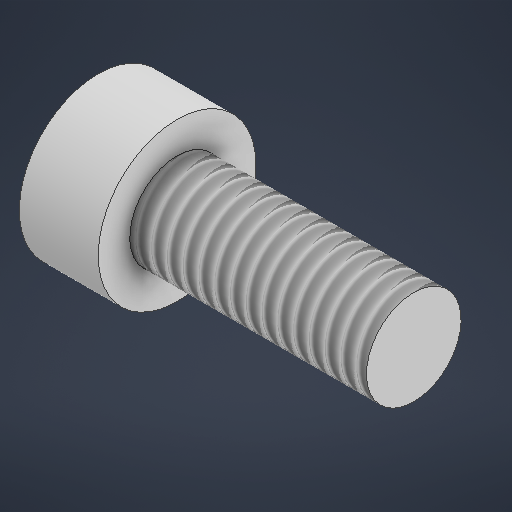
# Autodesk Inventor part: TORNILLO DE PRUEBA
Saved by Autodesk Inventor 2025 (Build 290162000, 162)
## iProperties
Created: 2026-02-06
Part Number: TORNILLO DE PRUEBA
Material: Genérico
Document SubType Name: Modeling
Designer: ROLANDO
Density: 1 g/cm^3
Appearance: Valor por defecto
Author: ROLANDO
Autodesk Inventor part; units mm, degrees
ref_plane "YZ Plane" through (0, 0, 0) normal (1, 0, 0) x (0, 1, 0)
ref_plane "XZ Plane" through (0, 0, 0) normal (0, 1, 0) x (-1, 0, 0)
ref_plane "XY Plane" through (0, 0, 0) normal (0, 0, 1) x (1, 0, 0)
sketch "Boceto1" plane through (0, 0, 0) normal (0, 0, 1) x (1, 0, 0)
  line L0 (-20, 0) -> (-20, 5)
  line L1 (-20, 5) -> (-15, 5)
  line L2 (-15, 5) -> (-15, 3)
  line L3 (-15, 3) -> (0, 3)
  line L4 (0, 3) -> (0, 0)
  line L5 (0, 0) -> (-20, 0)
  dimension "d0" = 3
  dimension "d1" = 5
  dimension "d2" = 5
  dimension "d6" = 20
  constraints: 12 end point, 4 perpendicular, 2 point on line, 1 horizontal, 1 vertical
  measures "d0" distance between parallel lines of L5 L3
  measures "d1" distance between parallel lines of L5 L1
  measures "d2" distance between parallel lines of L0 L2
  measures "d6" distance of L4.end L0.start
revolve "Revolución1" add sketch "Boceto1" angle 360 about axis through (0, 0, 0) along (-1, 0, 0)
thread "Rosca1" size "M6x1" class "6g" standard "ANSI Metric M Profile" full length
